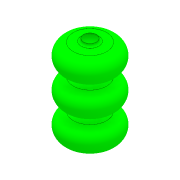
# Autodesk Inventor part: Lcavity949
Saved by Autodesk Inventor 2022.2 (Build 262287010, 287A)
## iProperties
Created: 2022-02-22
Part Number: Lcavity949
Material: Generic
Document SubType Name: Modeling
Designer: Josep
Density: 1 g/cm^3
Appearance: Cavity2
Author: Josep
Autodesk Inventor part; units mm, degrees
ref_plane "YZ Plane" through (0, 0, 0) normal (1, 0, 0) x (0, 1, 0)
ref_plane "XZ Plane" through (0, 0, 0) normal (0, 1, 0) x (-1, 0, 0)
ref_plane "XY Plane" through (0, 0, 0) normal (0, 0, 1) x (1, 0, 0)
sketch "Sketch1" plane through (0, 0, 0) normal (0, 1, 0) x (-1, 0, 0)
  arc A0 (-139.5416, 96.8345) -> (-139.5416, -96.8345) centre (-129.842, 0) ccw
  arc A1 (-54.0631, -125.308) -> (-73.8753, -103.4121) centre (-76.0686, -125.308) ccw
  line L0 (-139.5416, -96.8345) -> (-73.8753, -103.4121)
  line L1 (-139.5416, 96.8345) -> (-73.8753, 103.4121)
  arc A2 (-73.8753, 103.4121) -> (-54.0631, 125.308) centre (-76.0686, 125.308) ccw
  line L2 (-54.0631, -125.308) -> (-54.0631, -154.6881) construction
  line L3 (-54.0631, 125.308) -> (-54.0631, 163.9201) construction
  line L4 (0, -218.4097) -> (0, 227.6417) projected
  point P0 (0, 0)
  point P1 (-227.161, 0)
  dimension "d0" = 22.0055
  dimension "d2" = 250.616
  dimension "d3" = 227.161
  constraints: 8 end point, 7 point on circle, 6 tangent, 3 centre point, 2 vertical, 1 equal length, 1 equal radius, 1 horizontal alignment, 1 vertical alignment
  measures "d0" radius of A1
  measures "d2" distance of L3.start L2.start
  measures "d3" distance of point (0, 0) point (-227.161, 0)
surface revolve "RevolutionSrf1" sketch "Sketch1" angle 360 about axis through (0, 0, -10) along (0, 0, 1) shown no curves A1 L0 A0 L1 A2
thicken "Thicken1" operation new thickness 1 both sides no extend neighbours no toward (-0.5666588, -0.8236218, -0.0233465) faces at (-128.7428, -187.1239, -2.2721) (-114.3989, 50.251, -98.2961) (21.8674, -66.8564, -104.0607) (-114.3989, 50.251, 98.2961) (21.8674, -66.8564, 104.0607)
pattern_linear "Rectangular Pattern1" count 3 spacing 250.616 along (0, 0, 1) first direction both ways yes
body "Solid1"
body "Srf1"
